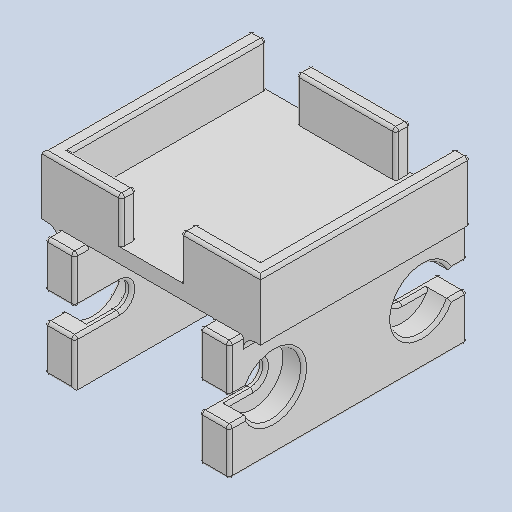
# Autodesk Inventor part: SMC-2000_case
Saved by Autodesk Inventor 2025.2 (Build 292293000, 293)
## iProperties
Created: 2025-07-30
Part Number: SMC-2000_case
Material: 일반
Document SubType Name: Modeling
Designer: jbhma
Density: 1 g/cm^3
Appearance: 기본값
Author: jbhma
Autodesk Inventor part; units mm, degrees
ref_plane "YZ Plane" through (0, 0, 0) normal (1, 0, 0) x (0, 1, 0)
ref_plane "XZ Plane" through (0, 0, 0) normal (0, 1, 0) x (-1, 0, 0)
ref_plane "XY Plane" through (0, 0, 0) normal (0, 0, 1) x (1, 0, 0)
sketch "스케치1" plane through (0, 0, 0) normal (0, 1, 0) x (-1, 0, 0)
  line L0 (36.75, -70.5) -> (-36.75, -70.5)
  line L1 (-36.75, -70.5) -> (-36.75, 0)
  line L2 (-36.75, 0) -> (36.75, 0)
  line L3 (36.75, 0) -> (36.75, -70.5)
  point P0 (0, 0)
  point P1 (0, 0)
  dimension "d0" = 70.5
  dimension "d1" = 73.5
  constraints: 8 end point, 2 parallel, 1 coincident, 1 horizontal, 1 midpoint, 1 perpendicular
  measures "d0" distance between parallel lines of L0 L2
  measures "d1" distance between parallel lines of L1 L3
extrude "돌출1" add sketch "스케치1" along normal blind 5
sketch "스케치2" plane through (0, 5, 0) normal (0, 1, 0) x (1, 0, 0)
  line L0 (-36.75, 0) -> (36.75, 0) projected
  line L1 (36.75, 0) -> (36.75, 70.5) projected
  line L2 (36.75, 70.5) -> (-36.75, 70.5) projected
  line L3 (-36.75, 70.5) -> (-36.75, 0) projected
  line L4 (-36.75, 70.5) -> (36.75, 70.5)
  line L5 (36.75, 70.5) -> (36.75, 0)
  line L6 (36.75, 0) -> (-36.75, 0)
  line L7 (-36.75, 0) -> (-36.75, 70.5)
  line L8 (-31.75, 65.5) -> (31.75, 65.5)
  line L9 (31.75, 65.5) -> (31.75, 5)
  line L10 (31.75, 5) -> (-31.75, 5)
  line L11 (-31.75, 5) -> (-31.75, 65.5)
  point P0 (0, 0)
  dimension "d4" = 5
  constraints: 16 end point, 2 parallel, 1 horizontal, 1 perpendicular, 3 other
  measures "d4" distance between parallel lines of L2 L8
extrude "돌출2" add sketch "스케치2" along normal blind 15
sketch "스케치3" plane through (-36.75, 0, 0) normal (0, 0, 1) x (1, 0, 0)
  line L0 (0, 0) -> (73.5, 0) projected
  line L1 (73.5, 0) -> (73.5, 20) projected
  line L2 (0, 20) -> (73.5, 20) projected
  line L3 (0, 0) -> (0, 20) projected
  line L4 (26.75, 20) -> (46.75, 20)
  line L5 (46.75, 20) -> (46.75, 5)
  line L6 (46.75, 5) -> (26.75, 5)
  line L7 (26.75, 5) -> (26.75, 20)
  point P0 (36.75, 0)
  point P1 (36.75, 20)
  dimension "d7" = 20
  dimension "d8" = 15
  constraints: 8 end point, 2 midpoint, 2 parallel, 1 horizontal, 1 perpendicular, 1 point on line
  measures "d7" distance of L5.end L6.end
  measures "d8" distance of L4.end L5.end
extrude "돌출3" cut sketch "스케치3" against normal blind 15 contours L2 L5 L6 L7
sketch "스케치4" plane through (36.75, 0, -70.5) normal (0, 0, -1) x (-1, 0, 0)
  line L0 (0, 0) -> (73.5, 0) projected
  line L1 (73.5, 0) -> (73.5, 20) projected
  line L2 (0, 20) -> (73.5, 20) projected
  line L3 (0, 0) -> (0, 20) projected
  line L4 (5, 20) -> (20, 20)
  line L5 (20, 20) -> (20, 5)
  line L6 (20, 5) -> (5, 5)
  line L7 (5, 5) -> (5, 20)
  line L8 (53.5, 20) -> (68.5, 20)
  line L9 (68.5, 20) -> (68.5, 5)
  line L10 (68.5, 5) -> (53.5, 5)
  line L11 (53.5, 5) -> (53.5, 20)
  point P0 (36.75, 0)
  point P1 (20, 20)
  dimension "d11" = 15
  dimension "d12" = 15
  dimension "d13" = 15
  dimension "d14" = 15
  dimension "d15" = 5
  dimension "d16" = 5
  constraints: 16 end point, 4 parallel, 2 horizontal, 2 perpendicular, 2 point on line
  measures "d11" distance of L5.end L6.end
  measures "d12" distance of L4.end L5.end
  measures "d13" distance of L9.end L10.end
  measures "d14" distance of L8.end L9.end
  measures "d15" distance between parallel lines of L3 L7
  measures "d16" distance between parallel lines of L1 L9
extrude "돌출4" cut sketch "스케치4" against normal blind 5 contours L2 L5 L6 L7 | L9 L10 L11 L2
sketch "스케치6" plane through (0, 0, 0) normal (0, -1, 0) x (1, 0, 0)
  line L0 (-36.75, 0) -> (36.75, 0) projected
  line L1 (-36.75, -70.5) -> (-36.75, 0) projected
  line L2 (36.75, -70.5) -> (-36.75, -70.5) projected
  line L3 (36.75, 0) -> (36.75, -70.5) projected
  line L4 (0, 0) -> (0, -70.5) construction
  line L5 (-36.75, -35.25) -> (36.75, -35.25) construction
  line L6 (-31, 4.75) -> (-21, 4.75)
  line L7 (-21, 4.75) -> (-21, -75.25)
  line L8 (-21, -75.25) -> (-31, -75.25)
  line L9 (-31, -75.25) -> (-31, 4.75)
  line L10 (21, 4.75) -> (31, 4.75)
  line L11 (31, 4.75) -> (31, -75.25)
  line L12 (31, -75.25) -> (21, -75.25)
  line L13 (21, -75.25) -> (21, 4.75)
  point P0 (-31, -35.25)
  dimension "d25" = 10
  dimension "d26" = 80
  dimension "d27" = 10
  dimension "d28" = 80
  dimension "d29" = 42
  dimension "d30" = 21
  constraints: 20 end point, 4 midpoint, 4 parallel, 2 horizontal, 2 perpendicular, 2 point on line
  measures "d25" distance of L7.end L8.end
  measures "d26" distance of L6.end L7.end
  measures "d27" distance of L11.end L12.end
  measures "d28" distance of L10.end L11.end
  measures "d29" distance between parallel lines of L13 L7
  measures "d30" distance between parallel lines of L4 L7
extrude "돌출6" add sketch "스케치6" along normal blind 40 contours L9 L6 L7 L0 | L0 L7 L2 L9 | L2 L7 L8 L9 | L13 L10 L11 L0 | L0 L11 L2 L13 | L2 L11 L12 L13
sketch "스케치7" plane through (31, 0, -70.5) normal (1, 0, 0) x (0, 0, -1)
  line L0 (4.75, 0) -> (0, 0) projected
  line L1 (-70.5, 0) -> (0, 0) projected
  line L2 (-70.5, 0) -> (-75.25, 0) projected
  line L3 (-75.25, 0) -> (-75.25, -40) projected
  line L4 (4.75, -40) -> (-75.25, -40) projected
  line L5 (4.75, 0) -> (4.75, -40) projected
  line L6 (-75.25, -20.074) -> (4.75, -20.074) construction
  arc A0 (-60.25, -24.324) -> (-60.25, -15.824) centre (-60.25, -20.074) ccw
  arc A1 (-10.25, -15.824) -> (-10.25, -24.324) centre (-10.25, -20.074) ccw
  line L7 (-75.25, -15.824) -> (-60.25, -15.824)
  line L8 (-60.25, -15.824) -> (-60.25, -24.324)
  line L9 (-60.25, -24.324) -> (-75.25, -24.324)
  line L10 (-75.25, -24.324) -> (-75.25, -15.824)
  line L11 (-10.25, -15.824) -> (4.75, -15.824)
  line L12 (4.75, -15.824) -> (4.75, -24.324)
  line L13 (4.75, -24.324) -> (-10.25, -24.324)
  line L14 (-10.25, -24.324) -> (-10.25, -15.824)
  dimension "d33" = 20.074
  dimension "d34" = 8.5
  dimension "d35" = 8.5
  dimension "d36" = 15
  dimension "d37" = 15
  constraints: 18 end point, 8 point on line, 4 parallel, 4 point on circle, 3 perpendicular, 2 centre point, 2 horizontal, 1 tangent
  measures "d33" distance between parallel lines of L6 L1
  measures "d34" diameter of A0
  measures "d35" diameter of A1
  measures "d36" distance from line of L3 A0.centre
  measures "d37" distance from line of L5 A1.centre
extrude "돌출7" cut sketch "스케치7" against normal blind 100 contours L5 L13 L14 L11 | L14 A1 | L7 L8 L9 L3 | A0 L8
sketch "스케치8" plane through (31, 0, -70.5) normal (1, 0, 0) x (0, 0, -1)
  line L0 (-10.25, -15.824) -> (4.75, -15.824) projected
  line L1 (4.75, 0) -> (4.75, -15.824) projected
  line L2 (4.75, 0) -> (0, 0) projected
  line L3 (-70.5, 0) -> (0, 0) projected
  line L4 (-70.5, 0) -> (-75.25, 0) projected
  line L5 (-75.25, 0) -> (-75.25, -15.824) projected
  line L6 (-75.25, -15.824) -> (-60.25, -15.824) projected
  arc A0 (-60.25, -24.324) -> (-60.25, -15.824) centre (-60.25, -20.074) ccw projected
  line L7 (-60.25, -24.324) -> (-75.25, -24.324) projected
  line L8 (-75.25, -24.324) -> (-75.25, -40) projected
  line L9 (4.75, -40) -> (-75.25, -40) projected
  line L10 (4.75, -24.324) -> (4.75, -40) projected
  line L11 (4.75, -24.324) -> (-10.25, -24.324) projected
  arc A1 (-10.25, -15.824) -> (-10.25, -24.324) centre (-10.25, -20.074) ccw projected
  arc A2 (-69.3019, -24.324) -> (-69.3019, -15.824) centre (-60.25, -20.074) ccw
  arc A3 (-1.1981, -15.824) -> (-1.1981, -24.324) centre (-10.25, -20.074) ccw
  dimension "d40" = 20
  dimension "d41" = 20
  constraints: 4 point on circle, 4 point on line, 2 centre point, 2 coincident
  measures "d40" diameter of A2
  measures "d41" diameter of A3
extrude "돌출8" cut sketch "스케치8" against normal blind 7 contours A1 L11 A3 L0 | L7 A0 L6 A2
sketch "스케치9" plane through (-31, 0, 0) normal (-1, 0, 0) x (0, 0, 1)
  line L0 (-75.25, -15.824) -> (-60.25, -15.824) projected
  arc A0 (-60.25, -24.324) -> (-60.25, -15.824) centre (-60.25, -20.074) ccw projected
  line L1 (-60.25, -24.324) -> (-75.25, -24.324) projected
  line L2 (-75.25, -24.324) -> (-75.25, -40) projected
  line L3 (4.75, -40) -> (-75.25, -40) projected
  line L4 (4.75, -24.324) -> (4.75, -40) projected
  line L5 (4.75, -24.324) -> (-10.25, -24.324) projected
  arc A1 (-10.25, -15.824) -> (-10.25, -24.324) centre (-10.25, -20.074) ccw projected
  line L6 (-10.25, -15.824) -> (4.75, -15.824) projected
  line L7 (4.75, 0) -> (4.75, -15.824) projected
  line L8 (4.75, 0) -> (0, 0) projected
  line L9 (-70.5, 0) -> (0, 0) projected
  line L10 (-70.5, 0) -> (-75.25, 0) projected
  line L11 (-75.25, 0) -> (-75.25, -15.824) projected
  arc A2 (-69.3019, -24.324) -> (-69.3019, -15.824) centre (-60.25, -20.074) ccw
  arc A3 (-1.1981, -15.824) -> (-1.1981, -24.324) centre (-10.25, -20.074) ccw
  point P0 (0, 0)
  dimension "d44" = 20
  dimension "d45" = 20
  constraints: 4 point on circle, 4 point on line, 2 centre point, 2 coincident
  measures "d44" diameter of A2
  measures "d45" diameter of A3
extrude "돌출9" cut sketch "스케치9" against normal blind 7 contours A2 L1 A0 L0 | L6 A1 L5 A3
fillet "모깎기1" radius 1 40 edges at (31, -7.912, 4.75) (26, 0, 4.75) (21, -7.912, 4.75) (26, -24.324, 4.75) (26, -15.824, 4.75) (21, -32.162, 4.75) (26, -40, 4.75) (31, -32.162, 4.75) (24, -20.074, -14.5) (24, -15.824, -5.724) (24, -24.324, -5.724) (31, -20.074, -20.25) (31, -15.824, 1.776) (31, -24.324, 1.776) (31, -20.074, -50.25) (24, -24.324, -64.776) (24, -15.824, -64.776) (24, -20.074, -56) (31, -15.824, -72.276) (31, -24.324, -72.276) (31, -32.162, -75.25) (26, -40, -75.25) (21, -32.162, -75.25) (21, -7.912, -75.25) (31, -7.912, -75.25) (26, -15.824, -75.25) (26, -24.324, -75.25) (26, 0, -75.25) (21, -20.074, -56) (21, -15.824, -67.75) (21, -24.324, -67.75) (21, -15.824, -2.75) (21, -24.324, -2.75) (21, -20.074, -14.5) (31, 0, 2.375) (21, 0, 2.375) (31, -40, -35.25) (21, -40, -35.25) (21, 0, -72.875) (31, 0, -72.875)
fillet "모깎기2" radius 1 39 edges at (-21, -15.824, -67.75) (-21, -24.324, -67.75) (-21, -20.074, -56) (-24, -15.824, -64.776) (-24, -24.324, -64.776) (-24, -20.074, -56) (-31, -20.074, -50.25) (-31, -7.912, -75.25) (-21, -7.912, -75.25) (-26, 0, -75.25) (-26, -15.824, -75.25) (-26, -24.324, -75.25) (-21, -32.162, -75.25) (-31, -32.162, -75.25) (-26, -40, -75.25) (-31, -15.824, -72.276) (-31, -24.324, -72.276) (-31, -20.074, -20.25) (-31, -15.824, 1.776) (-31, -24.324, 1.776) (-24, -20.074, -14.5) (-24, -15.824, -5.724) (-24, -24.324, -5.724) (-21, -20.074, -14.5) (-21, -15.824, -2.75) (-21, -24.324, -2.75) (-26, -24.324, 4.75) (-31, -7.912, 4.75) (-31, 0, 2.375) (-21, 0, 2.375) (-26, 0, 4.75) (-31, 0, -72.875) (-21, 0, -72.875) (-31, -40, -35.25) (-31, -32.162, 4.75) (-26, -15.824, 4.75) (-21, -7.912, 4.75) (-26, -40, 4.75) (-21, -32.162, 4.75)
fillet "모깎기3" radius 4 2 edges at (31, 0, -35.25) (-31, 0, -35.25)
fillet "모깎기4" radius 1 16 edges at (23.375, 20, 0) (-23.375, 20, 0) (-36.75, 20, -35.25) (-34.25, 20, -70.5) (0, 20, -70.5) (36.75, 20, -35.25) (31.75, 20, -37.75) (20.875, 20, -5) (-20.875, 20, -5) (-31.75, 20, -37.75) (0, 20, -65.5) (-16.75, 20, -68) (16.75, 20, -68) (34.25, 20, -70.5) (-10, 20, -2.5) (10, 20, -2.5)
fillet "모깎기5" radius 1 24 edges at (-10, 12, 0) (-10.2929, 19.7071, -0.2929) (-10.2929, 19.7071, -4.7071) (-10, 12, -5) (10.2929, 19.7071, -0.2929) (10, 12, 0) (10, 12, -5) (10.2929, 19.7071, -4.7071) (16.4571, 19.7071, -65.7929) (16.75, 12, -65.5) (16.4571, 19.7071, -70.2071) (16.75, 12, -70.5) (32.0429, 19.7071, -70.2071) (31.75, 12, -70.5) (36.4571, 19.7071, -70.2071) (36.75, 9.5, -70.5) (-16.4571, 19.7071, -65.7929) (-16.75, 12, -65.5) (-16.75, 12, -70.5) (-16.4571, 19.7071, -70.2071) (-32.0429, 19.7071, -70.2071) (-31.75, 12, -70.5) (-36.75, 9.5, -70.5) (-36.4571, 19.7071, -70.2071)
